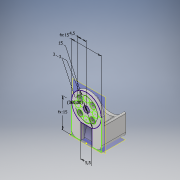
# Autodesk Inventor part: uchyt motoru
Saved by Autodesk Inventor 2018 (Build 220112000, 112)
## iProperties
Created: 2018-03-10
Part Number: uchyt motoru
Material: Všeobecné
Document SubType Name: Modeling
Designer: Kuba
Density: 1 g/cm^3
Appearance: Výchozí
Author: Kuba
Autodesk Inventor part; units mm, degrees
ref_plane "YZ Plane" through (0, 0, 0) normal (1, 0, 0) x (0, 1, 0)
ref_plane "XZ Plane" through (0, 0, 0) normal (0, 1, 0) x (-1, 0, 0)
ref_plane "XY Plane" through (0, 0, 0) normal (0, 0, 1) x (1, 0, 0)
sketch "Náčrt1" plane through (0, 0, 0) normal (0, 1, 0) x (-1, 0, 0)
  arc A0 (2.75, -6.9776) -> (-2.75, -6.9776) centre (0, 0) ccw
  line L0 (-7.5, 0) -> (-7.5, -15)
  line L1 (7.5, -15) -> (7.5, 0)
  line L2 (2.75, -6.9776) -> (-2.75, -6.9776)
  line L3 (-2.75, -6.9776) -> (-2.75, -15)
  line L4 (2.75, -15) -> (2.75, -6.9776)
  circle A1 centre (4.5, 0) radius 1.5
  circle A2 centre (0, 0) radius 1.5
  circle A3 centre (0, 4.5) radius 1.5
  circle A4 centre (-4.5, 0) radius 1.5
  circle A5 centre (0, -4.5) radius 1.5
  line L5 (-7.5, -15) -> (-2.75, -15)
  line L6 (2.75, -15) -> (7.5, -15)
  circle A6 centre (3.182, 3.182) radius 1.5
  circle A7 centre (0, 4.5) radius 1.5
  circle A8 centre (-3.182, 3.182) radius 1.5
  circle A9 centre (-4.5, 0) radius 1.5
  circle A10 centre (-3.182, -3.182) radius 1.5
  circle A11 centre (0, -4.5) radius 1.5
  circle A12 centre (3.182, -3.182) radius 1.5
  line L7 (-1.5, 0) -> (-3, 0)
  line L8 (-6, 0) -> (-7.5, 0)
  line L9 (7.5, 0) -> (6, 0)
  line L10 (3, 0) -> (1.5, 0)
  dimension "d0" = 15
  dimension "d1" = 3
  dimension "d2" = 3
  dimension "d5" = 360
  dimension "d7" = 4.5
  dimension "d8" = 5.5
  dimension "d9" = 15
  dimension "d10" = 15
  dimension "d13" = 360
  constraints: 22 end point, 13 centre point, 10 parallel, 9 point on circle, 5 horizontal, 5 perpendicular, 2 coincident, 26 other
  measures "d0" diameter of A0
  measures "d1" diameter of A1
  measures "d2" diameter of A2
  measures "d7" distance of point (0, 0) A1.centre
  measures "d8" distance of L2.start L2.end
  measures "d9" distance between parallel lines of L0 L1
  measures "d10" distance of L1.start L1.end
extrude "Vysunutí1" add sketch "Náčrt1" along normal blind 1.5 contours L2 A0 L8 A4 L7 A2 L10 A1 L9 | A0 L1 L6 L4 | L9 A1 L10 A2 L7 A4 L8 A0 | L3 L5 L0 A0 | A1 | A4 | A3 | A5
sketch "Náčrt2" plane through (0, 0, 0) normal (0, -1, 0) x (1, 0, 0)
  point P0 (0, 0)
ref_plane "Pracovní rovina1" through (0, 1.5, 0) normal (0, 1, 0) x (1, 0, 0)
sketch "Náčrt3" plane through (0, 1.5, 0) normal (0, 1, 0) x (1, 0, 0)
  arc A0 (7.5, 1.9526) -> (-7.5, 1.9526) centre (0, 0) ccw
  line L0 (-7.5, 15) -> (-7.5, 0) projected
  line L1 (7.5, 15) -> (2.75, 15) projected
  line L2 (7.5, 1.9526) -> (7.5, 15)
  line L3 (7.5, 15) -> (-7.5, 15)
  line L4 (-7.5, 15) -> (-7.5, 1.9526)
  dimension "d18" = 15.5
  constraints: 6 end point, 2 point on circle, 1 centre point, 1 coincident, 1 parallel, 1 point on line
  measures "d18" diameter of A0
extrude "Vysunutí2" add sketch "Náčrt3" along normal blind 11
ref_plane "Pracovní rovina2" through (-2.75, 0, -15) normal (0, 0, -1) x (-1, 0, 0)
sketch "Náčrt4" plane through (-2.75, 0, -15) normal (0, 0, -1) x (-1, 0, 0)
  line L0 (-5.5, 0) -> (-5.5, 1.5) projected
  line L1 (-5.5, 1.5) -> (0, 1.5)
  line L2 (0, 1.5) -> (0, 3.5)
  line L3 (0, 3.5) -> (-5.5, 3.5)
  line L4 (-5.5, 3.5) -> (-5.5, 1.5)
  point P0 (-2.75, 0)
  constraints: 8 end point, 2 parallel, 1 horizontal, 1 perpendicular
extrude "Vysunutí3" cut sketch "Náčrt4" against normal blind 9
fillet "Zaoblení1" radius 0.5 1 edges at (7.5, 7, -1.9526)
fillet "Zaoblení2" radius 0.5 1 edges at (-7.5, 7, -1.9526)
sketch "Náčrt5" plane through (-2.75, 0, -15) normal (0, 0, -1) x (-1, 0, 0)
  point P0 (-2.75, 0)
sketch "Náčrt6" plane through (-2.75, 0, -6.9776) normal (1, 0, 0) x (0, 0, -1)
  point P0 (-6.9776, 0)
sketch "Náčrt7" plane through (-2.75, 0, -6.9776) normal (1, 0, 0) x (0, 0, -1)
  point P0 (-6.9776, 0)
sketch "Náčrt8" plane through (-2.75, 0, -6.9776) normal (1, 0, 0) x (0, 0, -1)
  line L0 (8.0224, 1.4999) -> (1, 3.5)
  line L1 (8.0224, 3.5) -> (0.268, 3.5) projected
  line L2 (1, 3.5) -> (8.0224, 3.5)
  line L3 (8.0224, 3.5) -> (8.0224, 1.4999)
  point P0 (-6.9776, 0)
  constraints: 6 end point, 1 perpendicular
extrude "Vysunutí4" add sketch "Náčrt8" along normal blind 7
sketch "Náčrt9" plane through (-2.75, 0, -15) normal (0, 0, -1) x (-1, 0, 0)
  line L0 (0, 0) -> (0, 1.4999) projected
  line L1 (0, 0) -> (4.75, 0) projected
  line L2 (4.75, 0) -> (4.75, 12.5) projected
  line L3 (-10.25, 12.5) -> (4.75, 12.5) projected
  line L4 (-10.25, 0) -> (-10.25, 12.5) projected
  line L5 (-10.25, 0) -> (-5.5, 0) projected
  line L6 (-5.5, 0) -> (-5.5, 1.4999) projected
  line L7 (0, 1.4999) -> (-5.5, 1.4999) projected
  line L8 (-6, 4.4999) -> (0.5, 4.4999)
  line L9 (0.5, 4.4999) -> (0.5, 10.9999)
  line L10 (0.5, 10.9999) -> (-6, 10.9999)
  line L11 (-6, 10.9999) -> (-6, 4.4999)
  point P0 (-2.75, 0)
  dimension "d28" = 6.5
  dimension "d29" = 6.5
  dimension "d30" = 3
  dimension "d31" = 0.5
  constraints: 8 end point, 2 parallel, 1 horizontal, 1 perpendicular
  measures "d28" distance of L10.end L8.start
  measures "d29" distance of L9.end L10.end
  measures "d30" distance between parallel lines of L7 L8
  measures "d31" distance between parallel lines of L6 L11
extrude "Vysunutí5" cut sketch "Náčrt9" against normal blind 8 contours L11 L10 L9 L8
fillet "Zaoblení3" radius 0.5 1 edges at (0, 1.4999, -15)
fillet "Zaoblení4" radius 0.5 1 edges at (1.5, 1.5, 0)
fillet "Zaoblení5" radius 2.5 2 edges at (-7.5, 6.25, -15) (7.5, 6.25, -15)
fillet "Zaoblení6" radius 1 2 edges at (0, 3.5, -7.75) (0, 1.5, -6.9776)
equation "\"d9\" = d0"
equation "\"d29\" = d28"
equation "\"d31\" = -0.5 * d8 + 0.5 * d28"
